Autodesk Inventor part; units mm, degrees
(part 2 of 2)
  point P98 (33.9946, 372)
  point P99 (33.9946, 324)
  point P100 (33.9946, 340)
  point P101 (33.9946, 292)
  point P102 (33.9946, 308)
  point P103 (33.9946, 260)
  point P104 (33.9946, 276)
  point P105 (33.9946, 228)
  point P106 (33.9946, 244)
  point P107 (33.9946, 196)
  point P108 (33.9946, 212)
  point P109 (33.9946, 484)
  point P110 (33.9946, 500)
  point P111 (33.9946, 452)
  point P112 (33.9946, 468)
  point P113 (33.9946, 420)
  point P114 (33.9946, 436)
  point P115 (33.9946, 388)
  point P116 (33.9946, 404)
  point P117 (33.9946, 356)
  point P118 (33.9946, 372)
  point P119 (33.9946, 324)
  point P120 (33.9946, 340)
  point P121 (33.9946, 292)
  point P122 (33.9946, 308)
  point P123 (33.9946, 260)
  point P124 (33.9946, 276)
  point P125 (33.9946, 228)
  point P126 (33.9946, 244)
  point P127 (33.9946, 516)
  point P128 (33.9946, 532)
  point P129 (33.9946, 484)
  point P130 (33.9946, 500)
  point P131 (33.9946, 452)
  point P132 (33.9946, 468)
  point P133 (33.9946, 420)
  point P134 (33.9946, 436)
  point P135 (33.9946, 388)
  point P136 (33.9946, 404)
  point P137 (33.9946, 356)
  point P138 (33.9946, 372)
  point P139 (33.9946, 324)
  point P140 (33.9946, 340)
  point P141 (33.9946, 292)
  point P142 (33.9946, 308)
  point P143 (33.9946, 260)
  point P144 (33.9946, 276)
  point P145 (33.9946, 548)
  point P146 (33.9946, 564)
  point P147 (33.9946, 516)
  point P148 (33.9946, 532)
  point P149 (33.9946, 484)
  point P150 (33.9946, 500)
  point P151 (33.9946, 452)
  point P152 (33.9946, 468)
  point P153 (33.9946, 420)
  point P154 (33.9946, 436)
  point P155 (33.9946, 388)
  point P156 (33.9946, 404)
  point P157 (33.9946, 356)
  point P158 (33.9946, 372)
  point P159 (33.9946, 324)
  point P160 (33.9946, 340)
  point P161 (33.9946, 292)
  point P162 (33.9946, 308)
  point P163 (-128.5227, 600)
  point P164 (-86.745, 292)
  point P165 (-86.745, 308)
  point P166 (-86.745, 260)
  point P167 (-86.745, 276)
  point P168 (-86.745, 228)
  point P169 (-86.745, 244)
  point P170 (-86.745, 196)
  point P171 (-86.745, 212)
  point P172 (-86.745, 164)
  point P173 (-86.745, 180)
  point P174 (-86.745, 132)
  point P175 (-86.745, 148)
  point P176 (-86.745, 100)
  point P177 (-86.745, 116)
  point P178 (-86.745, 68)
  point P179 (-86.745, 84)
  point P180 (-86.745, 36)
  point P181 (-86.745, 52)
  point P182 (-86.745, 324)
  point P183 (-86.745, 340)
  point P184 (-86.745, 292)
  point P185 (-86.745, 308)
  point P186 (-86.745, 260)
  point P187 (-86.745, 276)
  point P188 (-86.745, 228)
  point P189 (-86.745, 244)
  point P190 (-86.745, 196)
  point P191 (-86.745, 212)
  point P192 (-86.745, 164)
  point P193 (-86.745, 180)
  point P194 (-86.745, 132)
  point P195 (-86.745, 148)
  point P196 (-86.745, 100)
  point P197 (-86.745, 116)
  point P198 (-86.745, 68)
  point P199 (-86.745, 84)
  dimension "d62" = 18
  dimension "d72" = 18
  dimension "d83" = 18
  dimension "d63" = 8
  dimension "d66" = 32
  dimension "d69" = 32
  dimension "d74" = 8
  dimension "d77" = 32
  dimension "d80" = 32
  dimension "d84" = 8
  dimension "d87" = 32
  dimension "d90" = 32
  constraints: 246 vertical, 81 vertical alignment, 30 end point, 9 midpoint, 6 parallel, 3 horizontal, 3 perpendicular, 1450 other
  measures "d63" distance from line of L6 point (33.995, 308)
  measures "d66" distance of point (33.995, 300) point (33.995, 268)
  measures "d69" distance of point (33.995, 300) point (33.995, 332)
  measures "d74" distance of point (-86.745, 300) point (-86.745, 308)
  measures "d77" distance of point (-86.745, 300) point (-86.745, 268)
  measures "d80" distance of point (-86.745, 300) point (-86.745, 332)
  measures "d84" distance from line of L21 point (-204.619, 308)
  measures "d87" distance of point (-204.619, 300) point (-204.619, 268)
  measures "d90" distance of point (-204.619, 300) point (-204.619, 332)
extrude "Extrusión5" cut sketch "Boceto3" along normal mid plane 32.5 contours E0 L6 | L6 E0 | E1 | E2 | E3 | E4 | E5 | E6 | E7 | E8 | E9 | E18 | E27 | E36 | E45 | E54 | E63 | E72 | E81 L13 | L13 E81 | E82 | E83 | E84 | E85 | E86 | E87 | E88 | E89 | E90 | E99 | E108 | E117 | E126 | E135 | E144 | E153 | E162 L21 | L21 E162 | E163 | E164 | E165 | E166 | E167 | E168 | E169 | E170 | E171 | E180 | E189 | E198 | E207 | E216 | E225 | E234
equation "\"Radio_pliegue\" = Grosor"
equation "\"Anchura_desahogo_plegado\" = Grosor"
equation "\"Profundidad_desahogo_plegado\" = 0.5 * Grosor"
equation "\"Tamaño_destalonado\" = 4 * Grosor"
equation "\"Remanente_mínimo\" = 2 * Grosor"
equation "\"Radiodetransición\" = Radio_pliegue"
equation "\"Tamaño_de_radio_de_Jacobi\" = Grosor"
equation "\"TamañoSeparación\" = Grosor"
equation "\"Grosor\" = 4"
